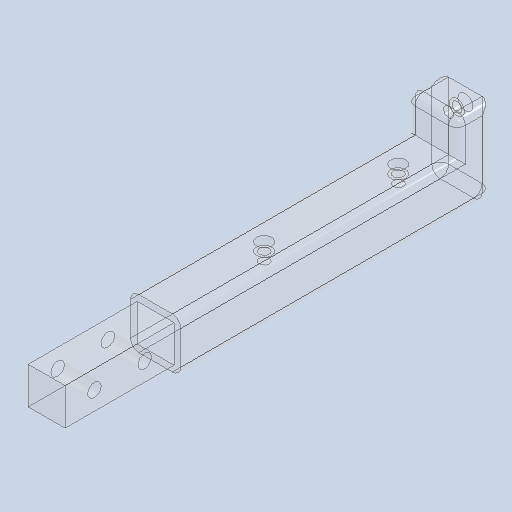
# Autodesk Inventor part: L
Saved by Autodesk Inventor 2025.3 (Build 293356000, 356)
## iProperties
Created: 2026-04-18
Part Number: L
Material: PCTG 20%
Document SubType Name: Modeling
Designer: ksawe
Density: 1.541 g/cm^3
Appearance: Polycarbonate - Clear(1)
Author: ksawe
Autodesk Inventor part; units mm, degrees
ref_plane "YZ Plane" through (0, 0, 0) normal (1, 0, 0) x (0, 1, 0)
ref_plane "XZ Plane" through (0, 0, 0) normal (0, 1, 0) x (-1, 0, 0)
ref_plane "XY Plane" through (0, 0, 0) normal (0, 0, 1) x (1, 0, 0)
sketch "Sketch1" plane through (0, 0, 0) normal (0, 1, 0) x (-1, 0, 0)
  line L0 (15, 124.835) -> (-15, 124.835)
  line L1 (-15, 124.835) -> (-15, -124.835)
  line L2 (-15, -124.835) -> (15, -124.835)
  line L3 (15, -124.835) -> (15, 124.835)
  line L4 (15, 124.835) -> (-15, -124.835) construction
  line L5 (-15, 124.835) -> (15, -124.835) construction
  point P0 (0, 0)
  dimension "d0" = 30
  dimension "d1" = 249.67
  constraints: 12 end point, 2 midpoint, 2 parallel, 1 horizontal, 1 perpendicular
  measures "d0" distance of L2.end L1.end
  measures "d1" distance of L0.end L1.end
extrude "Extrusion1" add sketch "Sketch1" along normal blind 30
sketch "Sketch2" plane through (0, 30, 0) normal (0, 1, 0) x (1, 0, 0)
  line L0 (15, 124.835) -> (-15, 124.835) projected
  line L1 (-15, 124.835) -> (-15, -124.835) projected
  line L2 (15, 124.835) -> (-15, 124.835)
  line L3 (-15, 124.835) -> (-15, 104.835)
  line L4 (-15, 104.835) -> (15, 104.835)
  line L5 (15, 104.835) -> (15, 124.835)
  point P0 (0, 0)
  dimension "d4" = 20
  constraints: 8 end point, 2 parallel, 1 horizontal, 1 perpendicular, 1 point on line
  measures "d4" distance of L4.end L0.start
extrude "Extrusion2" add sketch "Sketch2" along normal blind 20
sketch "Sketch3" plane through (-15, 0, 124.835) normal (0, 0, 1) x (1, 0, 0)
  line L0 (0, 0) -> (30, 0) projected
  line L1 (30, 0) -> (30, 30) projected
  line L2 (0, 30) -> (30, 30) projected
  line L3 (0, 0) -> (0, 30) projected
  line L4 (4, 26) -> (26, 26)
  line L5 (26, 26) -> (26, 4)
  line L6 (26, 4) -> (4, 4)
  line L7 (4, 4) -> (4, 26)
  point P0 (15, 0)
  dimension "d7" = 4
  constraints: 8 end point, 3 other
  measures "d7" distance between parallel lines of L3 L7
extrude "Extrusion3" cut sketch "Sketch3" against normal blind 65
sketch "Sketch4" plane through (15, 0, -124.835) normal (0, 0, -1) x (-1, 0, 0)
  line L0 (0, 50) -> (30, 50) projected
  line L1 (30, 0) -> (30, 50) projected
  point P0 (15, 0)
  point P1 (15, 42)
  dimension "d10" = 8
  dimension "d11" = 15
  measures "d10" distance from line of L0 point (15, 42)
  measures "d11" distance from line of L1 point (15, 42)
hole "Hole1" at (0, 42, -124.835) direction (0, 0, 1) diameter 6 depth 10 tip angle 118 counterbore diameter 9 counterbore depth 5
sketch "Sketch5" plane through (11, 4, 124.835) normal (1, 0, 0) x (0, 0, -1)
  circle A0 centre (17.5, 11) radius 4
  circle A1 centre (47.5, 11) radius 4
  line L0 (65, 26) -> (65, -4) projected
  line L1 (0, 0) -> (0, 22) projected
  line L2 (0, 0) -> (65, 0) projected
  point P0 (124.835, -4)
  point P1 (65, 11)
  point P2 (0, 11)
  dimension "d19" = 8
  dimension "d20" = 8
  dimension "d21" = 30
  dimension "d23" = 17.5
  constraints: 2 centre point, 2 horizontal alignment, 2 midpoint
  measures "d19" diameter of A0
  measures "d20" diameter of A1
  measures "d21" distance of A1.centre A0.centre
  measures "d23" distance from line of L1 A0.centre
extrude "Extrusion4" cut sketch "Sketch5" against normal through all
fillet "Fillet1" radius 5 12 edges at (15, 25, -124.835) (-15, 25, -124.835) (0, 0, -124.835) (15, 0, -32.5) (-15, 0, -32.5) (15, 30, -22.5) (-15, 30, -22.5) (15, 40, -104.835) (-15, 40, -104.835) (0, 50, -104.835) (15, 50, -114.835) (-15, 50, -114.835)
sketch "Sketch6" plane through (0, 30, 0) normal (0, 1, 0) x (1, 0, 0)
  line L0 (-10, 104.835) -> (10, 104.835) projected
  line L1 (-10, -59.835) -> (-10, 104.835) projected
  point P0 (0, 0)
  point P1 (0, 84.835)
  point P2 (0, 4.835)
  dimension "d28" = 20
  dimension "d36" = 100
  dimension "d37" = 10
  dimension "d38" = 10
  measures "d28" distance from line of L0 point (0, 84.835)
  measures "d36" distance from line of L0 point (0, 4.835)
  measures "d37" distance from line of L1 point (0, 4.835)
  measures "d38" distance from line of L1 point (0, 84.835)
hole "Hole2" at (0, 30, -4.835) at (0, 30, -84.835) direction (0, -1, 0) diameter 6 depth 10 tip angle 118 counterbore diameter 9 counterbore depth 5
body "Solid1"
